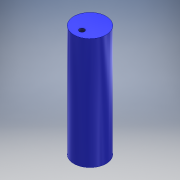
# Autodesk Inventor part: Tubo Soporte para Corte
Saved by Autodesk Inventor 2018 (Build 220112000, 112)
## iProperties
Created: 2019-05-21
Part Number: Tubo Soporte para Corte
Material: Generic
Document SubType Name: Modeling
Designer: Ivan
Density: 1 g/cm^3
Appearance: 12in Running - Burgundy
Author: Ivan
Autodesk Inventor part; units mm, degrees
ref_plane "YZ Plane" through (0, 0, 0) normal (1, 0, 0) x (0, 1, 0)
ref_plane "XZ Plane" through (0, 0, 0) normal (0, 1, 0) x (-1, 0, 0)
ref_plane "XY Plane" through (0, 0, 0) normal (0, 0, 1) x (1, 0, 0)
sketch "Sketch1" plane through (0, 0, 0) normal (0, 0, 1) x (1, 0, 0)
  circle A0 centre (0, 0) radius 6.35
  dimension "d2" = 12.7
  constraints: 2 coincident, 1 centre point
  measures "d2" diameter of A0
extrude "Extrusion1" add sketch "Sketch1" along normal mid plane 44
sketch "Sketch2" plane through (0, 0, 22) normal (0, 0, 1) x (1, 0, 0)
  circle A0 centre (0, -3.175) radius 1
  point P0 (0, 0)
  dimension "d3" = 2
  dimension "d4" = 3.175
  constraints: 1 centre point, 1 vertical alignment
  measures "d3" diameter of A0
  measures "d4" distance of point (0, 0) A0.centre
hole "Hole1" at (0, -3.175, 22) direction (0, 0, -1) diameter 2 depth 6
mirror "Mirror1" about plane through (0, 0, 0) normal (0, 0, 1) of "Hole1"
thread "Thread1" size "M2x0.4" class "6H" standard "ANSI Metric M Profile" full length
thread "Thread2" size "M2x0.4" class "6H" standard "ANSI Metric M Profile" full length
body "Solid1"
